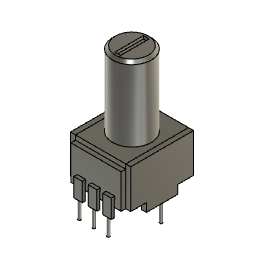
POT_2.54mmp_H13mm_3pin (Autodesk Fusion 360 design; units mm, degrees)
Autodesk Fusion 360 part; units mm, degrees
note: some values were not read from the file. Set by a fixed rule: which sketch regions a step uses.
sketch "スケッチ1" plane through (0, 0, 0) normal (0, 0, 1) x (1, 0, 0)
  line L0 (-4.4, -5.5) -> (4.4, -5.5)
  line L1 (4.4, -5.5) -> (4.4, 5.5)
  line L2 (4.4, 5.5) -> (-4.4, 5.5)
  line L3 (-4.4, 5.5) -> (-4.4, -5.5)
  line L4 (0, 8.9294) -> (0, 2.0706) construction
  line L5 (6.4126, 0) -> (2.3874, 0) construction
  line L6 (0, 1.75) -> (0, 22.5)
  line L7 (1.75, 0) -> (22.5, 0)
  dimension "d1" = 8.8
  dimension "d2" = 11
  constraint horizontal L0
  constraint vertical L1
  constraint horizontal L2
  constraint vertical L3
  constraint vertical L4
  constraint horizontal L5
  constraint midpoint L1 L5
  constraint midpoint L2 L4
  constraint collinear L4 L6
  constraint collinear L5 L7
  measures "d1" distance of L0.start L0.end
  measures "d2" distance of L0.start L2.end
extrude "押し出し1" add sketch "スケッチ1" along normal blind 6.8 makes body 1
sketch "スケッチ2" plane through (0, 0, 6.8) normal (0, 0, 1) x (-1, 0, 0)
  line L0 (4.4, -5.5) -> (4.4, 5.5)
  line L1 (4.4, 5.5) -> (-4.4, 5.5)
  line L2 (-4.4, 5.5) -> (-4.4, -5.5)
  line L3 (-4.4, -5.5) -> (4.4, -5.5)
  circle A0 centre (0, 0) radius 3.4
  line L4 (0, -3.1614) -> (0, 14.1614) construction
  line L5 (14.4499, 0) -> (-5.6499, 0) construction
  dimension "d5" = 6.8
  constraint vertical L4
  constraint midpoint L1 L4
  constraint coincident A0.centre L4
  constraint horizontal L5
  constraint midpoint L0 L5
  constraint coincident A0.centre L5
  measures "d5" diameter of A0
extrude "押し出し2" add sketch "スケッチ2" along normal blind 13 contours A0 bodies 1
sketch "スケッチ3" plane through (0, 0, 19.8) normal (0, 0, 1) x (-1, 0, 0)
  circle A0 centre (0, 0) radius 3.4
  line L0 (0.5, -2.5) -> (-0.5, -2.5)
  line L1 (-0.5, -2.5) -> (-0.5, 2.5)
  line L2 (-0.5, 2.5) -> (0.5, 2.5)
  line L3 (0.5, 2.5) -> (0.5, -2.5)
  line L4 (0, -4.5952) -> (0, 4.5952) construction
  line L5 (-4.2273, 0) -> (4.2273, 0) construction
  dimension "d8" = 5
  dimension "d9" = 1
  constraint horizontal L0
  constraint vertical L1
  constraint horizontal L2
  constraint vertical L3
  constraint vertical L4
  constraint perpendicular L1 L5
  constraint coincident A0.centre L5
  constraint coincident A0.centre L4
  constraint midpoint L4 L5
  constraint symmetric L1 L3 L4
  constraint symmetric L0 L2 L5
  measures "d8" distance of L0 L2
  measures "d9" distance of L0.start L0.end
extrude "押し出し3" cut sketch "スケッチ3" against normal blind 0.5 contours L0 L1 L2 L3 bodies 1
sketch "スケッチ4" plane through (0, -5.5, 0) normal (0, -1, 0) x (1, 0, 0)
  line L0 (-4.4, 0) -> (4.4, 0)
  line L1 (4.4, 0) -> (4.4, 6.8)
  line L2 (4.4, 6.8) -> (-4.4, 6.8)
  line L3 (-4.4, 6.8) -> (-4.4, 0)
  line L4 (4.4, 0) -> (-4.4, 0)
  line L5 (-4.4, 0) -> (-4.4, 6)
  line L6 (-4.4, 6) -> (4.4, 6)
  line L7 (4.4, 6) -> (4.4, 0)
  dimension "d12" = 6
  constraint horizontal L4
  constraint vertical L5
  constraint horizontal L6
  constraint vertical L7
  constraint coincident L3 L5.end
  constraint coincident L0.end L1.start
  measures "d12" distance of L4 L6
extrude "押し出し4" add sketch "スケッチ4" along normal blind 0.8 contours L0 L1 L3 L4 L5 L6 L7 bodies 1
sketch "スケッチ5" plane through (0, -6.3, 0) normal (0, -1, 0) x (1, 0, 0)
  line L0 (4.4, 6) -> (-4.4, 6)
  line L1 (-4.4, 6) -> (-4.4, 0)
  line L2 (-4.4, 0) -> (4.4, 0)
  line L3 (4.4, 0) -> (4.4, 6)
  line L4 (-0.75, 1.75) -> (0.75, 1.75)
  line L5 (0.75, 1.75) -> (0.75, 1.25)
  line L6 (0.75, 1.25) -> (-0.75, 1.25)
  line L7 (-0.75, 1.25) -> (-0.75, 1.75)
  line L8 (0, -0.7679) -> (0, 0.7679) construction
  line L9 (0, 2.3784) -> (0, 0.1216) construction
  dimension "d15" = 1.5
  dimension "d16" = 0.5
  dimension "d18" = 1.25
  constraint horizontal L4
  constraint vertical L5
  constraint horizontal L6
  constraint vertical L7
  constraint vertical L8
  constraint midpoint L2 L8
  constraint vertical L9
  constraint midpoint L6 L9
  constraint collinear L8 L9
  measures "d15" distance of L4.start L4.end
  measures "d16" distance of L4.start L6.end
  measures "d18" distance of L2 L6
extrude "押し出し5" add sketch "スケッチ5" along normal blind 0.6 contours L4 L5 L6 L7 bodies 1
sketch "スケッチ6" plane through (0, 0, 1.25) normal (0, 0, -1) x (1, 0, 0)
  line L0 (-0.75, 6.3) -> (0.75, 6.3)
  line L1 (0.75, 6.3) -> (0.75, 6.9)
  line L2 (0.75, 6.9) -> (-0.75, 6.9)
  line L3 (-0.75, 6.9) -> (-0.75, 6.3)
  line L4 (-0.75, 6.9) -> (0.75, 6.9)
  line L5 (0.75, 6.9) -> (0.75, 6.4)
  line L6 (0.75, 6.4) -> (-0.75, 6.4)
  line L7 (-0.75, 6.4) -> (-0.75, 6.9)
  dimension "d21" = 0.5
  constraint horizontal L4
  constraint vertical L5
  constraint horizontal L6
  constraint vertical L7
  constraint coincident L1 L5.end
  constraint coincident L2.end L3.start
  measures "d21" distance of L2.end L6.end
extrude "押し出し6" add sketch "スケッチ6" along normal blind 2.75 contours L1 L2 L3 L4 L5 L6 L7 bodies 1
sketch "スケッチ7" plane through (0, 0, -1.5) normal (0, 0, -1) x (1, 0, 0)
  line L0 (-0.75, 6.4) -> (0.75, 6.4)
  line L1 (0.75, 6.4) -> (0.75, 6.9)
  line L2 (0.75, 6.9) -> (-0.75, 6.9)
  line L3 (-0.75, 6.9) -> (-0.75, 6.4)
  circle A0 centre (0, 6.65) radius 0.25
  line L4 (0, 7.0161) -> (0, 6.7839) construction
  dimension "d24" = 0.5
  constraint tangent L2 A0
  constraint vertical L4
  constraint midpoint L2 L4
  constraint coincident A0.centre L4
  measures "d24" diameter of A0
extrude "押し出し7" add sketch "スケッチ7" along normal blind 3 contours A0 bodies 1
pattern_linear "R パターン1" count 3 spacing 2.54 along (1, 0, 0) both ways of "押し出し5", "押し出し6", "押し出し7"
sketch "スケッチ8" plane through (-4.4, 0, 0) normal (-1, 0, 0) x (0, 1, 0)
  line L0 (-5.5, -6.8) -> (5.5, -6.8)
  line L1 (5.5, -6.8) -> (5.5, 0)
  line L2 (5.5, 0) -> (-5.5, 0)
  line L3 (-5.5, 0) -> (-5.5, -6.8)
  line L4 (5.5, 0) -> (-6.3, 0)
  line L5 (-6.3, 0) -> (-6.3, -6)
  line L6 (-6.3, -6) -> (-5.5, -6)
  line L7 (-5.5, -6) -> (-5.5, -6.8)
  line L8 (-5.5, -6.8) -> (5.5, -6.8)
  line L9 (5.5, -6.8) -> (5.5, 0)
  line L10 (2.75, 0) -> (-2.75, 0)
  line L11 (-2.75, 0) -> (-2.75, 1.5)
  line L12 (-2.75, 1.5) -> (2.75, 1.5)
  line L13 (2.75, 1.5) -> (2.75, 0)
  line L14 (0, 0.7349) -> (0, 2.2651) construction
  line L15 (0, -7.7985) -> (0, -5.8015) construction
  dimension "d31" = 11
  dimension "d32" = 6.8
  dimension "d35" = 5.5
  dimension "d36" = 1.5
  constraint horizontal L0
  constraint vertical L1
  constraint horizontal L2
  constraint vertical L3
  constraint coincident L0.start L3.end
  constraint horizontal L10
  constraint vertical L11
  constraint horizontal L12
  constraint vertical L13
  constraint coincident L4 L10.start
  constraint perpendicular L12 L14
  constraint perpendicular L0 L15
  constraint midpoint L0 L15
  constraint midpoint L12 L14
  constraint collinear L14 L15
  measures "d31" distance of L0.start L0.end
  measures "d32" distance of L0.start L2.end
  measures "d35" distance of L10.start L10.end
  measures "d36" distance of L10.end L11.end
extrude "押し出し8" add sketch "スケッチ8" along normal blind 0.88 separate body contours L0 L1 L2 L3 L4 L7 L8 L9 L10 | L2 L4 L10 L11 L12 L13 makes body 2
sketch "スケッチ9" plane through (0, 0, -1.5) normal (0, 0, -1) x (1, 0, 0)
  line L0 (-4.4, -2.75) -> (-4.4, 2.75)
  line L1 (-4.4, 2.75) -> (-5.28, 2.75)
  line L2 (-5.28, 2.75) -> (-5.28, -2.75)
  line L3 (-5.28, -2.75) -> (-4.4, -2.75)
  circle A0 centre (-5.08, 0) radius 0.25
  line L4 (-2.54, 1.2313) -> (-2.54, -1.0687) construction
  point P0 (-2.54, 6.4)
  dimension "d37" = 0.5
  dimension "d39" = 2.54
  constraint vertical L4
  constraint coincident L4 P0
  measures "d37" diameter of A0
  measures "d39" distance of A0.centre L4
extrude "押し出し9" add sketch "スケッチ9" along normal blind 3 contours L2 A0 | L2 A0 bodies 2
mirror "ミラー1" about plane through (0, 0, 0) normal (1, 0, 0) of "押し出し8", "押し出し9" makes body 3
chamfer "面取り1" distance 0.5 angle 45 1 edges at (3.1699, 1.2295, 19.8) on bodies 1
